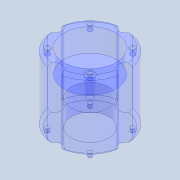
# Autodesk Inventor part: cpd_lowrcf_0.7_p3_v1
Saved by Autodesk Inventor 2021.2 (Build 252289000, 289)
## iProperties
Created: 2021-12-08
Part Number: cpd_lowrcf_0.7_p3_v1
Material: Generic
Document SubType Name: Modeling
Designer: tomos
Density: 1 g/cm^3
Appearance: Clear - Blue
Author: tomos
Autodesk Inventor part; units mm, degrees
ref_plane "YZ Plane" through (0, 0, 0) normal (1, 0, 0) x (0, 1, 0)
ref_plane "XZ Plane" through (0, 0, 0) normal (0, 1, 0) x (-1, 0, 0)
ref_plane "XY Plane" through (0, 0, 0) normal (0, 0, 1) x (1, 0, 0)
sketch "Sketch1" plane through (0, 0, 0) normal (0, 0, 1) x (1, 0, 0)
  line L0 (0, 0) -> (0, 19.4488) construction
  line L1 (0, 0) -> (15.8946, 0) construction
  line L2 (1.0783, 9) -> (1.5923, 16)
  line L3 (1.0783, 9) -> (6.5, 9)
  line L4 (6.5, 9) -> (6.5, 0)
  line L5 (6.5, 0) -> (12.5, 0)
  line L6 (12.5, 0) -> (12.5, 24)
  line L7 (1.5923, 16) -> (9, 16)
  line L8 (9, 16) -> (9, 24)
  line L9 (9, 24) -> (12.5, 24)
  line L10 (1.0783, 9) -> (1.0049, 8) construction
  line L11 (1.0049, 8) -> (0.7849, 8) construction
  line L12 (1.5923, 16) -> (2.5, 28.36) construction
  line L13 (2.5, 28.36) -> (1.5, 28.36) construction
  line L14 (0.7849, 8) -> (0.4645, 1) construction
  line L15 (0.4645, 1) -> (0.2, 1) construction
  line L16 (0.2, 1) -> (1.5, 28.36) construction
  line L17 (0, 6.7) -> (1.1563, 6.7) construction
  line L18 (0.4708, 6.7) -> (0.4708, 8.6077) construction
  dimension "d1" = 12.5
  dimension "d2" = 6.5
  dimension "d7" = 9
  dimension "d8" = 9
  dimension "d45" = 24
  dimension "d46" = 8
  dimension "d47" = 4.2
  dimension "d49" = 20.36
  dimension "d50" = 2.5
  dimension "d51" = 2.62
  dimension "d53" = 0.22
  dimension "d54" = 7
  dimension "d55" = 0.2
  dimension "d56" = 1
  dimension "d57" = 5.7
  dimension "d58" = 2.3
  constraints: 38 end point, 6 horizontal, 5 perpendicular, 5 point on line, 2 collinear, 2 vertical
  measures "d1" distance between parallel lines of L6 L0
  measures "d2" distance between parallel lines of L4 L0
  measures "d7" distance between parallel lines of L3 L1
  measures "d8" distance between parallel lines of L8 L0
  measures "d45" distance between parallel lines of L1 L9
  measures "d46" distance between parallel lines of L9 L7
  measures "d47" angle of L12 L0
  measures "d49" distance between parallel lines of L13 L11
  measures "d50" distance from line of L12.end L0
  measures "d51" angle of L14 L0
  measures "d53" distance of L10.end L11.end
  measures "d54" distance between parallel lines of L15 L11
  measures "d55" distance from line of L0 L15.end
  measures "d56" distance of L12.end L13.end
  measures "d57" distance between parallel lines of L17 L15
  measures "d58" distance between parallel lines of L3 L17
revolve "Revolution1" add sketch "Sketch1" angle 360 about axis through (0, 0, 0) along (0, 1, 0)
chamfer "Chamfer2" distance 1 angle 45 2 edges at (-12.5, 0, 0) (-12.5, 24, 0)
sketch "Sketch2" plane through (0, 0, 0) normal (0, -1, 0) x (1, 0, 0)
  circle A0 centre (0, 0) radius 1.0783 construction
  circle A1 centre (0, 0) radius 10.5 construction
  circle A2 centre (0, 0) radius 1.5923 construction
  line L0 (0, 0) -> (19.4803, 0) construction
  line L1 (0, 0) -> (20.4554, -20.4554) construction
  circle A3 centre (7.4246, -7.4246) radius 0.75
  circle A4 centre (0, 0) radius 12.5
  circle A5 centre (12.5, 0) radius 2.5
  point P0 (12.25, 2.4875)
  point P1 (12.25, -2.4875)
  dimension "d19" = 21
  dimension "d23" = 25
  dimension "d20" = 45
  dimension "d21" = 1.5
  dimension "d22" = 5
  constraints: 4 end point, 2 centre point, 2 coincident, 2 point on line, 1 horizontal, 6 other
  measures "d20" angle of L1 L0
  measures "d21" diameter of A3
  measures "d22" diameter of A5
extrude "Extrusion1" cut sketch "Sketch2" against normal through all contours A4 A5 picked at (11.6823, -0.4803)
extrude "Extrusion2" add sketch "Sketch2" along normal blind 1.5 contours A3
chamfer "Chamfer3" distance 0.35 angle 45 1 edges at (6.6746, -1.5, -7.4246)
pattern_circular "Circular Pattern1" count 4 over 360 about axis through (0, -10, 0) along (0, 1, 0) of "Extrusion1", "Extrusion2", "Chamfer3"
sketch "Sketch3" plane through (12.5, 24, 0) normal (0, 1, 0) x (1, 0, 0)
  circle A0 centre (-12.5, 0) radius 1.0783 construction
  line L0 (-12.5, 0) -> (0.4785, 0) construction
  line L1 (-12.5, 0) -> (-1.2806, -11.2194) construction
  circle A1 centre (-12.5, 0) radius 10.5 construction
  circle A2 centre (-5.0754, -7.4246) radius 0.8
  dimension "d34" = 21
  dimension "d35" = 45
  dimension "d36" = 1.6
  constraints: 4 end point, 2 centre point, 2 coincident, 1 horizontal
  measures "d34" diameter of A1
  measures "d35" angle of L0 L1
  measures "d36" diameter of A2
extrude "Extrusion3" cut sketch "Sketch3" against normal blind 2
chamfer "Chamfer4" distance 0.25 angle 45 1 edges at (6.6246, 24, 7.4246)
pattern_circular "Circular Pattern2" count 4 over 360 about axis through (0, -10, 0) along (0, 1, 0) of "Extrusion3", "Chamfer4"
equation "\"d57\" = cutpipette_length"
equation "\"cutpipette_length\" = 5.7"
body "Solid1"
